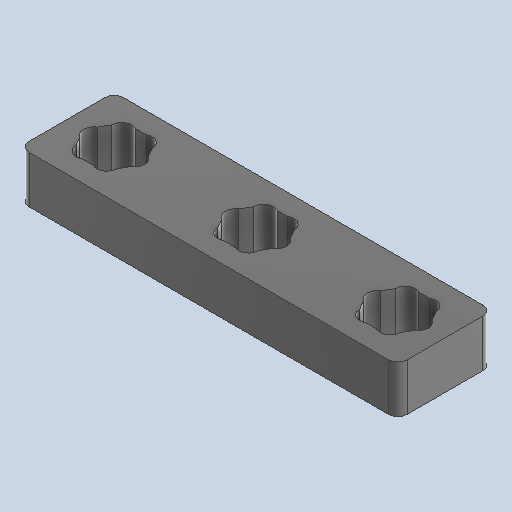
# Autodesk Inventor part: Trunk_abdomen_spacer
Saved by Autodesk Inventor 2022.4 (Build 264492000, 492)
## iProperties
Created: 2021-09-11
Part Number: Trunk_abdomen_spacer
Material: アセタール樹脂、黒
Document SubType Name: Modeling
Designer: Masato
Density: 1.425 g/cm^3
Appearance: 滑らか - 黒
Mass: 2.23775 g
Surface Area: 14.1946 cm^2
Volume: 1.57035 cm^3
Description: POM T5
Author: Masato Kubotera
Autodesk Inventor part; units mm, degrees
ref_plane "YZ Plane" through (0, 0, 0) normal (1, 0, 0) x (0, 1, 0)
ref_plane "XZ Plane" through (0, 0, 0) normal (0, 1, 0) x (-1, 0, 0)
ref_plane "XY Plane" through (0, 0, 0) normal (0, 0, 1) x (1, 0, 0)
derived "Trunk_vertical_frame_03.ipt"
sketch "スケッチ1" plane through (0, 0, 0) normal (0, 0, 1) x (1, 0, 0)
  circle A0 centre (0, 0) radius 11
  line L0 (1, 13.5) -> (28, 13.5) construction
  line L1 (28, 13.5) -> (28, -13.5) construction
  line L2 (28, -13.5) -> (1, -13.5) construction
  line L3 (1, -13.5) -> (1, 13.5) construction
  line L4 (1, 13.5) -> (28, -13.5) construction
  line L5 (28, 13.5) -> (1, -13.5) construction
  line L6 (-12, 16) -> (39.5, 16) construction
  line L7 (39.5, 16) -> (39.5, -16) construction
  line L8 (39.5, -16) -> (-12, -16) construction
  line L9 (-12, -16) -> (-12, 16) construction
  line L10 (-12, 16) -> (39.5, -16) construction
  line L11 (39.5, 16) -> (-12, -16) construction
  circle A1 centre (1, 13.5) radius 1.35
  arc A2 (0, 16) -> (-12, 10.583) centre (0, 0) ccw construction
  line L12 (-12, 0) -> (39.5, 0)
  circle A3 centre (28, 13.5) radius 1.35
  arc A4 (-12, -10.583) -> (0, -16) centre (0, 0) ccw construction
  circle A5 centre (28, -13.5) radius 1.35
  circle A6 centre (1, -13.5) radius 1.35
  arc A7 (0, 16.05) -> (-12.05, 10.6019) centre (0, 0) ccw
  line L13 (0, 16.05) -> (39.55, 16.05)
  line L14 (39.55, 16.05) -> (39.55, 13.3)
  line L15 (-12.05, 10.6019) -> (-12.05, 0)
  arc A8 (-11.5146, 11.1811) -> (-12.05, 9.86) centre (-11.0677, 10.2309) ccw
  line L16 (-12.05, 10.6019) -> (-11.0677, 10.2309) construction
  arc A9 (39.55, 14.5651) -> (38.0651, 16.05) centre (38.8075, 15.3075) ccw
  line L17 (38.8075, 15.3075) -> (39.55, 16.05) construction
  arc A10 (38.0651, -16.05) -> (39.55, -14.5651) centre (38.8075, -15.3075) ccw
  line L18 (-12.05, -10.6019) -> (-12.05, 0)
  arc A11 (-12.05, -9.86) -> (-11.5146, -11.1811) centre (-11.0677, -10.2309) ccw
  arc A12 (-12.05, -10.6019) -> (0, -16.05) centre (0, 0) ccw
  line L19 (0, -16.05) -> (39.55, -16.05)
  line L20 (39.55, 13.3) -> (42.05, 13.3)
  line L21 (42.05, 13.3) -> (42.05, -1.8)
  line L22 (42.05, -1.8) -> (39.55, -1.8)
  line L23 (39.55, -1.8) -> (39.55, -14.5651)
  line L24 (39.5, 13.25) -> (42, 13.25) construction
  line L25 (42, 13.25) -> (42, -1.75) construction
  line L26 (42, -1.75) -> (39.5, -1.75) construction
  line L27 (42, 5.75) -> (39.5, 5.75) construction
  arc A13 (42.05, 11.8151) -> (40.5651, 13.3) centre (41.3075, 12.5575) ccw
  line L28 (41.3075, 12.5575) -> (42.05, 13.3) construction
  arc A14 (40.5651, -1.8) -> (42.05, -0.3151) centre (41.3075, -1.0575) ccw
  circle A15 centre (-15.5, 19) radius 1.6
  line L29 (-18, 22) -> (-13, 22) construction
  line L30 (-13, 22) -> (-13, -10.5) construction
  line L31 (-13, -10.5) -> (-18, -10.5) construction
  line L32 (-18, -10.5) -> (-18, 22) construction
  line L33 (-18, 22) -> (-13, -10.5) construction
  line L34 (-13, 22) -> (-18, -10.5) construction
  line L35 (-18, 5.75) -> (-13, 5.75) construction
  line L36 (-15.5, 22) -> (-15.5, -10.5) construction
  line L37 (-18, 13.25) -> (-15.5, 13.25) construction
  line L38 (-15.5, 13.25) -> (-15.5, -1.75) construction
  line L39 (-15.5, -1.75) -> (-18, -1.75) construction
  line L40 (-18, 13.25) -> (-15.5, -1.75) construction
  line L41 (-15.5, 13.25) -> (-18, -1.75) construction
  line L42 (-15.45, -1.8) -> (-18.05, -1.8)
  line L43 (-18.05, -1.8) -> (-18.05, 13.3)
  line L44 (-18.05, 13.3) -> (-15.45, 13.3)
  line L45 (-15.45, 13.3) -> (-15.45, -1.8)
  line L46 (-15.45, -1.8) -> (-18.05, 13.3) construction
  line L47 (-18.05, -1.8) -> (-15.45, 13.3) construction
  line L48 (-16.75, 13.3) -> (-16.75, -1.8) construction
  arc A16 (-18.05, 13.3) -> (-18.05, 11.2) centre (-18.05, 12.25) ccw
  arc A17 (-15.45, 11.2) -> (-15.45, 13.3) centre (-15.45, 12.25) ccw
  arc A18 (-18.05, 0.3) -> (-18.05, -1.8) centre (-18.05, -0.75) ccw
  arc A19 (-15.45, -1.8) -> (-15.45, 0.3) centre (-15.45, -0.75) ccw
  circle A20 centre (-15.5, -7.5) radius 1.6
  line L49 (14.5, 16) -> (14.5, -16) construction
  circle A21 centre (42, 19) radius 1.6
  line L50 (39.5, 22) -> (44.5, 22) construction
  line L51 (44.5, 22) -> (44.5, -10.5) construction
  line L52 (44.5, -10.5) -> (39.5, -10.5) construction
  line L53 (39.5, 22) -> (44.5, -10.5) construction
  line L54 (44.5, 22) -> (39.5, -10.5) construction
  line L55 (42, 22) -> (42, -10.5) construction
  circle A22 centre (42, -7.5) radius 1.6
  line L56 (-12, -18.25) -> (27, -18.25) construction
  line L57 (27, -18.25) -> (27, -23.25) construction
  line L58 (27, -23.25) -> (-12, -23.25) construction
  line L59 (-12, -23.25) -> (-12, -18.25) construction
  line L60 (-12, -18.25) -> (27, -23.25) construction
  line L61 (27, -18.25) -> (-12, -23.25) construction
  line L62 (-3, -20.75) -> (18, -20.75) construction
  line L63 (18, -20.75) -> (18, -18.25) construction
  line L64 (-3, -18.25) -> (-3, -20.75) construction
  line L65 (-3, -20.75) -> (18, -18.25) construction
  line L66 (18, -20.75) -> (-3, -18.25) construction
  line L67 (-12, -20.75) -> (27, -20.75) construction
  line L68 (7.5, -18.25) -> (7.5, -23.25) construction
  line L69 (-3.05, -18.2) -> (18.05, -18.2)
  line L70 (18.05, -18.2) -> (18.05, -20.8)
  line L71 (18.05, -20.8) -> (-3.05, -20.8)
  line L72 (-3.05, -20.8) -> (-3.05, -18.2)
  line L73 (-3.05, -18.2) -> (18.05, -20.8) construction
  line L74 (18.05, -18.2) -> (-3.05, -20.8) construction
  circle A23 centre (-8, -20.75) radius 1.6
  circle A24 centre (23, -20.75) radius 1.6
  arc A25 (-0.95, -18.2) -> (-3.05, -18.2) centre (-2, -18.2) ccw
  arc A26 (18.05, -18.2) -> (15.95, -18.2) centre (17, -18.2) ccw
  line L75 (-3.05, -19.5) -> (18.05, -19.5) construction
  arc A27 (-3.05, -20.8) -> (-0.95, -20.8) centre (-2, -20.8) ccw
  arc A28 (15.95, -20.8) -> (18.05, -20.8) centre (17, -20.8) ccw
  circle A29 centre (-8, 20.75) radius 1.6
  line L76 (18.05, 20.8) -> (-3.05, 20.8)
  line L77 (-3.05, 19.5) -> (18.05, 19.5) construction
  line L78 (-3, 18.25) -> (-3, 20.75) construction
  line L79 (18, 20.75) -> (-3, 18.25) construction
  line L80 (-3, 20.75) -> (18, 18.25) construction
  line L81 (-3.05, 20.8) -> (-3.05, 18.2)
  line L82 (-3.05, 18.2) -> (18.05, 20.8) construction
  line L83 (-3.05, 18.2) -> (18.05, 18.2)
  arc A30 (-3.05, 18.2) -> (-0.95, 18.2) centre (-2, 18.2) ccw
  line L84 (18.05, 18.2) -> (-3.05, 20.8) construction
  line L85 (-12, 23.25) -> (-12, 18.25) construction
  arc A31 (-0.95, 20.8) -> (-3.05, 20.8) centre (-2, 20.8) ccw
  line L86 (7.5, 18.25) -> (7.5, 23.25) construction
  line L87 (-3, 20.75) -> (18, 20.75) construction
  line L88 (-12, 20.75) -> (27, 20.75) construction
  line L89 (27, 23.25) -> (-12, 23.25) construction
  line L90 (-12, 18.25) -> (27, 18.25) construction
  line L91 (-12, 18.25) -> (27, 23.25) construction
  line L92 (27, 18.25) -> (-12, 23.25) construction
  line L93 (27, 18.25) -> (27, 23.25) construction
  arc A32 (15.95, 18.2) -> (18.05, 18.2) centre (17, 18.2) ccw
  circle A33 centre (23, 20.75) radius 1.6
  line L94 (18, 20.75) -> (18, 18.25) construction
  line L95 (18.05, 18.2) -> (18.05, 20.8)
  arc A34 (18.05, 20.8) -> (15.95, 20.8) centre (17, 20.8) ccw
  line L96 (-18, 28.25) -> (44.5, 28.25)
  line L97 (-18, 28.25) -> (-23, 22)
  line L98 (44.5, 28.25) -> (47.5, 22)
  line L99 (-23, 22) -> (-23, -2.875)
  line L100 (47.5, 22) -> (47.5, -18.25)
  line L101 (47.5, -18.25) -> (37, -33.25)
  line L102 (-23, -2.875) -> (-33.5, -16)
  line L103 (-33.5, -16) -> (-33.5, -89)
  line L104 (37, -33.25) -> (37, -68.125)
  line L105 (37, -68.125) -> (23, -97)
  line L106 (23, -97) -> (-17, -97)
  line L107 (-17, -97) -> (-33.5, -89)
  circle A35 centre (-12, -92) radius 1.6
  circle A36 centre (3, -92) radius 1.6
  line L108 (-17, -97) -> (-17, -87)
  line L109 (-17, -87) -> (23, -87)
  line L110 (23, -87) -> (23, -97)
  line L111 (-17, -92) -> (23, -92) construction
  line L112 (3, -87) -> (3, -97) construction
  circle A37 centre (18, -92) radius 1.6
  circle A38 centre (-13.5, -54.25) radius 1.6
  line L113 (-23.5, -58.25) -> (27, -58.25)
  line L114 (27, -58.25) -> (27, -77)
  line L115 (27, -77) -> (-23.5, -77)
  line L116 (-23.5, -77) -> (-23.5, -58.25)
  line L117 (-23.5, -33.25) -> (27, -33.25)
  line L118 (27, -33.25) -> (27, -50.25)
  line L119 (27, -50.25) -> (-23.5, -50.25)
  line L120 (-23.5, -50.25) -> (-23.5, -33.25)
  circle A39 centre (-13.5, -54.25) radius 4 construction
  arc A40 (-11.4334, -94.8) -> (-9.8584, -93.8907) centre (-10.9084, -93.8907) ccw
  line L121 (-9.2918, -92.9093) -> (-9.8584, -93.8907)
  arc A41 (-9.2918, -92.9093) -> (-9.2918, -91.0907) centre (-9.8168, -92) ccw
  line L122 (-9.8584, -90.1093) -> (-9.2918, -91.0907)
  arc A42 (-9.8584, -90.1093) -> (-11.4334, -89.2) centre (-10.9084, -90.1093) ccw
  line L123 (-12.5666, -89.2) -> (-11.4334, -89.2)
  arc A43 (-12.5666, -89.2) -> (-14.1416, -90.1093) centre (-13.0916, -90.1093) ccw
  line L124 (-14.7082, -91.0907) -> (-14.1416, -90.1093)
  arc A44 (-14.7082, -91.0907) -> (-14.7082, -92.9093) centre (-14.1832, -92) ccw
  line L125 (-14.1416, -93.8907) -> (-14.7082, -92.9093)
  arc A45 (-14.1416, -93.8907) -> (-12.5666, -94.8) centre (-13.0916, -93.8907) ccw
  line L126 (-11.4334, -94.8) -> (-12.5666, -94.8)
  arc A46 (5.7082, -92.9093) -> (5.7082, -91.0907) centre (5.1832, -92) ccw
  line L127 (5.1416, -90.1093) -> (5.7082, -91.0907)
  line L128 (5.7082, -92.9093) -> (5.1416, -93.8907)
  arc A47 (3.5666, -94.8) -> (5.1416, -93.8907) centre (4.0916, -93.8907) ccw
  arc A48 (5.1416, -90.1093) -> (3.5666, -89.2) centre (4.0916, -90.1093) ccw
  line L129 (2.4334, -89.2) -> (3.5666, -89.2)
  arc A49 (2.4334, -89.2) -> (0.8584, -90.1093) centre (1.9084, -90.1093) ccw
  line L130 (0.2918, -91.0907) -> (0.8584, -90.1093)
  arc A50 (0.2918, -91.0907) -> (0.2918, -92.9093) centre (0.8168, -92) ccw
  line L131 (0.8584, -93.8907) -> (0.2918, -92.9093)
  arc A51 (0.8584, -93.8907) -> (2.4334, -94.8) centre (1.9084, -93.8907) ccw
  line L132 (3.5666, -94.8) -> (2.4334, -94.8)
  arc A52 (20.7082, -92.9093) -> (20.7082, -91.0907) centre (20.1832, -92) ccw
  line L133 (20.1416, -90.1093) -> (20.7082, -91.0907)
  line L134 (20.7082, -92.9093) -> (20.1416, -93.8907)
  arc A53 (18.5666, -94.8) -> (20.1416, -93.8907) centre (19.0916, -93.8907) ccw
  arc A54 (20.1416, -90.1093) -> (18.5666, -89.2) centre (19.0916, -90.1093) ccw
  line L135 (17.4334, -89.2) -> (18.5666, -89.2)
  arc A55 (17.4334, -89.2) -> (15.8584, -90.1093) centre (16.9084, -90.1093) ccw
  line L136 (15.2918, -91.0907) -> (15.8584, -90.1093)
  arc A56 (15.2918, -91.0907) -> (15.2918, -92.9093) centre (15.8168, -92) ccw
  line L137 (15.8584, -93.8907) -> (15.2918, -92.9093)
  arc A57 (15.8584, -93.8907) -> (17.4334, -94.8) centre (16.9084, -93.8907) ccw
  line L138 (18.5666, -94.8) -> (17.4334, -94.8)
  point P0 (14.5, 0)
  point P1 (-15.5, 5.75)
  point P2 (-16.75, 5.75)
  point P3 (14.5, 0)
  point P4 (42, 5.75)
  point P5 (42, 5.75)
  point P6 (7.5, -20.75)
  point P7 (7.5, -19.5)
  point P8 (7.5, -19.5)
  point P9 (7.5, -19.5)
  point P10 (7.5, -19.5)
  point P11 (7.5, 20.75)
  point P12 (7.5, 19.5)
  point P13 (7.5, 19.5)
  point P14 (7.5, 19.5)
  point P15 (7.5, 19.5)
  point P16 (-10.3834, -94.8)
  point P17 (-8.7668, -92)
  point P18 (-10.3834, -89.2)
  point P19 (-13.6166, -89.2)
  point P20 (-13.6166, -89.2)
  point P21 (-15.2332, -92)
  point P22 (-13.6166, -94.8)
  point P23 (-15.2332, -92)
  point P24 (-8.7668, -92)
  point P25 (3, -92)
  point P26 (6.2332, -92)
  point P27 (6.2332, -92)
  point P28 (4.6166, -89.2)
  point P29 (4.6166, -94.8)
  point P30 (3, -92)
  point P31 (3, -92)
  point P32 (1.3834, -89.2)
  point P33 (1.3834, -89.2)
  point P34 (-0.2332, -92)
  point P35 (-0.2332, -92)
  point P36 (1.3834, -94.8)
  point P37 (18, -92)
  point P38 (21.2332, -92)
  point P39 (21.2332, -92)
  point P40 (19.6166, -89.2)
  point P41 (19.6166, -94.8)
  point P42 (18, -92)
  point P43 (18, -92)
  point P44 (16.3834, -89.2)
  point P45 (16.3834, -89.2)
  point P46 (14.7668, -92)
  point P47 (14.7668, -92)
  point P48 (16.3834, -94.8)
  point P49 (15.8584, -90.1093)
  point P50 (0.8584, -90.1093)
  point P51 (-14.1416, -90.1093)
  point P52 (-0.95, 20.8)
  point P53 (15.95, 20.8)
  point P54 (15.95, 18.2)
  point P55 (15.95, -20.8)
  point P56 (-0.95, -20.8)
  point P57 (15.95, -18.2)
  point P58 (-18.05, 0.3)
  point P59 (-15.45, 0.3)
  point P60 (42.05, -0.3151)
  point P61 (40.5651, -1.8)
extrude "押し出し1" add sketch "スケッチ1" along normal blind 5 contours L108 L109 L110 L106
fillet "フィレット1" radius 1 4 edges at (-17, -87, 2.5) (-17, -97, 2.5) (23, -97, 2.5) (23, -87, 2.5)
